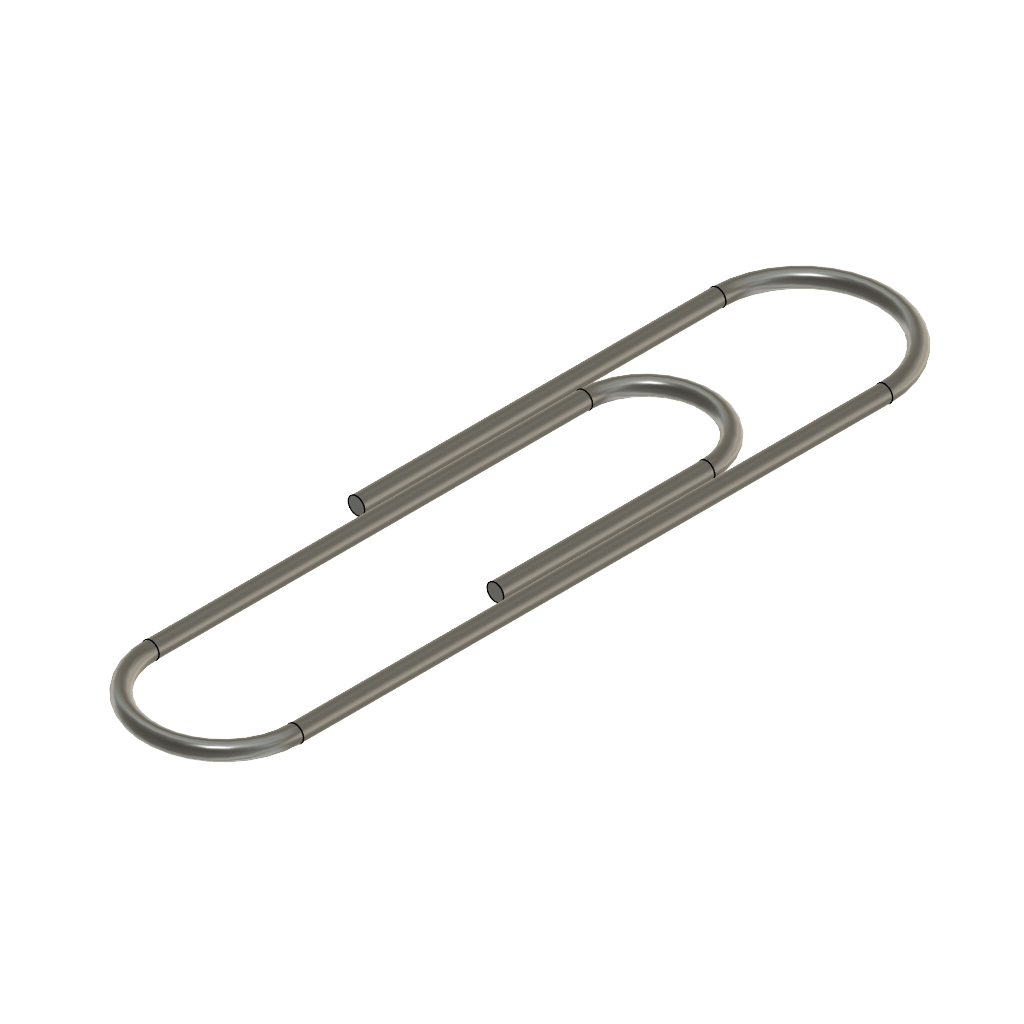
Paper Clip (Autodesk Fusion 360 design; units mm, degrees)
part number: 2026-09-10-12-01-48-744
Autodesk Fusion 360 part; units mm, degrees
sketch "Sweep path" plane through (0, 0, 0) normal (0, 0, 1) x (1, 0, 0)
  line L0 (0, 0) -> (0, 16.25)
  line L1 (0, 16.25) -> (7.5, 16.25) construction
  line L2 (7.5, 16.25) -> (7.5, -10.25)
  line L3 (7.5, -10.25) -> (1, -10.25) construction
  line L4 (1, -10.25) -> (1, 9.25)
  line L5 (1, 9.25) -> (6.5, 9.25) construction
  line L6 (6.5, 9.25) -> (6.5, -0.25)
  arc A0 (7.5, 16.25) -> (0, 16.25) centre (3.75, 16.25) ccw
  arc A1 (6.5, 9.25) -> (1, 9.25) centre (3.75, 9.25) ccw
  arc A2 (1, -10.25) -> (7.5, -10.25) centre (4.25, -10.25) ccw
  constraint coincident L0.start origin
  constraint vertical L0
  constraint perpendicular L0 L1
  constraint perpendicular L1 L2
  constraint perpendicular L2 L3
  constraint perpendicular L3 L4
  constraint perpendicular L4 L5
  constraint perpendicular L3 L6
  constraint tangent L0 A0
  constraint tangent L4 A1
  constraint tangent L2 A2
sketch "Sweep profile" plane through (0, 0, 0) normal (0, 1, 0) x (1, 0, 0)
  circle A0 centre (0, 0) radius 0.375
  dimension "d8" = 0.75
  constraint coincident A0.centre origin
  measures "d8" diameter of A0
sweep "Sweep1" add profiles "Sweep profile" path "Sweep path" along L0 A0 L2 A2 L4 A1 L6 section 1
